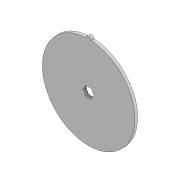
# Autodesk Inventor part: circle
Saved by Autodesk Inventor 2020 (Build 240168000, 168)
## iProperties
Created: 2021-06-15
Part Number: circle
Material: Generic
Document SubType Name: Modeling
Designer: Aidan Lee
Density: 1 g/cm^3
Appearance: Default
Author: Aidan Lee
Autodesk Inventor part; units mm, degrees
ref_plane "YZ Plane" through (0, 0, 0) normal (1, 0, 0) x (0, 1, 0)
ref_plane "XZ Plane" through (0, 0, 0) normal (0, 1, 0) x (-1, 0, 0)
ref_plane "XY Plane" through (0, 0, 0) normal (0, 0, 1) x (1, 0, 0)
sketch "Sketch1" plane through (0, 0, 0) normal (0, 0, 1) x (1, 0, 0)
  circle A0 centre (0, 0) radius 50
  circle A1 centre (0, 50) radius 2.75
  point P0 (-2.749, 49.9244)
  point P1 (2.749, 49.9244)
  dimension "d0" = 100
  dimension "d1" = 5.5
  constraints: 1 centre point, 1 coincident, 1 vertical alignment, 3 other
  measures "d1" diameter of A1
extrude "Extrusion1" add sketch "Sketch1" along normal blind 3
sketch "Sketch2" plane through (0, 0, 3) normal (0, 0, 1) x (1, 0, 0)
  arc A0 (-2.749, 49.9244) -> (2.749, 49.9244) centre (0, 0) ccw projected
  line L0 (-5.7735, 0) -> (-2.8868, 5)
  line L1 (-2.8868, 5) -> (2.8868, 5)
  line L2 (2.8868, 5) -> (5.7735, 0)
  line L3 (5.7735, 0) -> (2.8868, -5)
  line L4 (2.8868, -5) -> (-2.8868, -5)
  line L5 (-2.8868, -5) -> (-5.7735, 0)
  arc A1 (2.749, 49.9244) -> (-2.749, 49.9244) centre (0, 50) ccw construction
  line L6 (0, 0) -> (0, 50) construction
  dimension "d8" = 10
  constraints: 14 end point, 1 coincident, 1 perpendicular, 1 vertical, 13 other
  measures "d8" distance between parallel lines of L4 L1
extrude "Extrusion2" cut sketch "Sketch2" against normal through all
body "Solid1"
